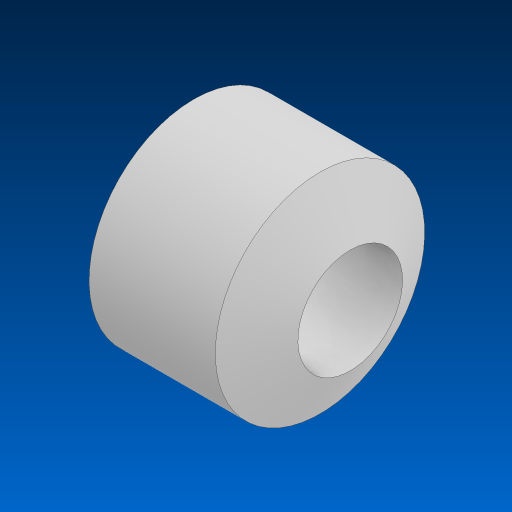
# Autodesk Inventor part: HUDSON-1-37
Saved by Autodesk Inventor 2023 (Build 270158000, 158)
## iProperties
Created: 2024-11-02
Part Number: HUDSON-1-37
Material: Generic
Document SubType Name: Modeling
Designer: CABALLERO
Density: 1 g/cm^3
Appearance: Default
Author: CABALLERO
Autodesk Inventor part; units mm, degrees
ref_plane "YZ Plane" through (0, 0, 0) normal (1, 0, 0) x (0, 1, 0)
ref_plane "XZ Plane" through (0, 0, 0) normal (0, 1, 0) x (-1, 0, 0)
ref_plane "XY Plane" through (0, 0, 0) normal (0, 0, 1) x (1, 0, 0)
sketch "Sketch1" plane through (0, 0, 0) normal (0, 0, 1) x (1, 0, 0)
  line L0 (-4.5, -5) -> (4.5, -5)
  line L1 (4.5, -5) -> (4.5, 2.5)
  line L2 (3.0566, 5) -> (-2.9701, 5)
  line L3 (-4.5, 2.3502) -> (-4.5, -5)
  line L4 (-4.5, -5) -> (4.5, 5) construction
  line L5 (-4.5, 0) -> (4.5, 0)
  line L6 (-4.5, 0) -> (-4.5, 2.5)
  line L7 (-4.5, 2.5) -> (-2.9701, 5)
  line L8 (4.5, 0) -> (4.5, 2.5)
  line L9 (4.5, 2.5) -> (3.0566, 5)
  line L10 (-4.5, -2.5) -> (4.5, -2.5)
  line L11 (4.5, -2.5) -> (4.5, 2.5)
  line L12 (4.5, 2.5) -> (-4.5, 2.5)
  line L13 (-4.5, 2.5) -> (-4.5, -2.5)
  line L14 (-4.5, -2.5) -> (4.5, 2.5) construction
  line L15 (4.5, -2.5) -> (-4.5, 2.5) construction
  point P0 (0, 0)
  dimension "d3" = 2.5
  dimension "d4" = 2.5
  dimension "d5" = 30
  constraints: 32 end point, 4 parallel, 3 midpoint, 3 point on line, 2 horizontal, 2 perpendicular
  measures "d3" distance of L5.start L6.end
  measures "d4" distance of L1.end L5.end
  measures "d5" angle of L1 L9
revolve "Revolution1" add sketch "Sketch1" angle 360 about axis through (-4.5, 0, 0) along (1, 0, 0) contours L12 L7 L2 L9
body "Solid1"
